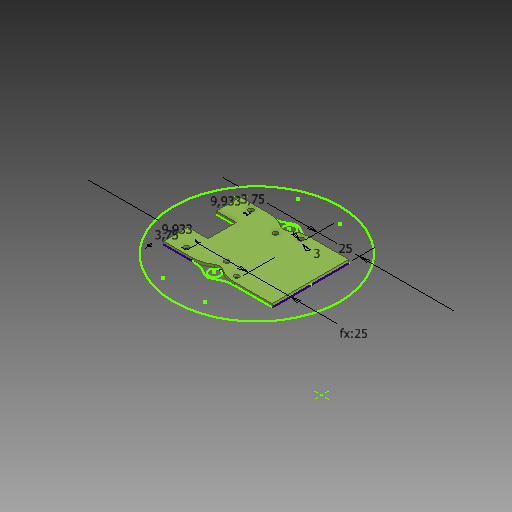
# Autodesk Inventor part: openMV_board
Saved by Autodesk Inventor 2020 (Build 240168000, 168)
## iProperties
Created: 2024-09-29
Part Number: openMV_board
Material: Типовые
Document SubType Name: Modeling
Designer: Ivan
Density: 1 g/cm^3
Appearance: Оливково-зеленый
Author: Ivan
Autodesk Inventor part; units mm, degrees
ref_plane "YZ Plane" through (0, 0, 0) normal (1, 0, 0) x (0, 1, 0)
ref_plane "XZ Plane" through (0, 0, 0) normal (0, 1, 0) x (-1, 0, 0)
ref_plane "XY Plane" through (0, 0, 0) normal (0, 0, 1) x (1, 0, 0)
sketch "Эскиз1" plane through (0, 0, 0) normal (0, 1, 0) x (-1, 0, 0)
  circle A0 centre (22.9, 3.75) radius 1.5
  circle A1 centre (53.2667, -35.05) radius 1.5
  circle A2 centre (22.9, -35.05) radius 1.5
  circle A3 centre (33.4, -38.2774) radius 3.3
  circle A4 centre (33.4, 6.9774) radius 3.3
  circle A5 centre (53.2667, 3.75) radius 1.5
  line L0 (63.2, -24.15) -> (51.2, -24.15)
  line L1 (51.2, -24.15) -> (51.2, -7.15)
  line L2 (51.2, -7.15) -> (63.2, -7.15)
  line L3 (63.2, -7.15) -> (63.2, 7.5)
  line L4 (63.2, 7.5) -> (46.0869, 7.5)
  arc A6 (35.969, 10.672) -> (46.0869, 7.5) centre (46.0869, 25.2227) ccw
  arc A7 (35.969, 10.672) -> (30.831, 10.672) centre (33.4, 6.9774) ccw
  arc A8 (20.7131, 7.5) -> (30.831, 10.672) centre (20.7131, 25.2227) ccw
  line L5 (20.7131, 7.5) -> (-2.1, 7.5)
  line L6 (-2.1, 7.5) -> (-2.1, -38.8)
  line L7 (-2.1, -38.8) -> (20.7131, -38.8)
  arc A9 (30.831, -41.972) -> (20.7131, -38.8) centre (20.7131, -56.5227) ccw
  arc A10 (30.831, -41.972) -> (35.969, -41.972) centre (33.4, -38.2774) ccw
  arc A11 (46.0869, -38.8) -> (35.969, -41.972) centre (46.0869, -56.5227) ccw
  line L8 (46.0869, -38.8) -> (63.2, -38.8)
  line L9 (63.2, -38.8) -> (63.2, -24.15)
  circle A12 centre (30.5522, -15.6437) radius 50
  line L10 (53.2667, -35.05) -> (22.9, -35.05)
  line L11 (53.2667, 3.75) -> (22.9, 3.75)
  point P0 (0, 0)
  point P1 (-2.1, -15.65)
  point P2 (0, 0)
  point P3 (-63.2, 38.8)
  point P4 (63.2, -38.8)
  dimension "d7" = 3.75
  dimension "d8" = 3.75
  dimension "d9" = 9.9333
  dimension "d10" = 9.9333
  dimension "d11" = 25
  dimension "d12" = 25
  dimension "d13" = 3
  constraints: 24 end point, 13 centre point, 12 point on circle, 3 equal radius, 2 horizontal, 8 other
  measures "d7" distance from line of L8 L10.start
  measures "d8" distance from line of L4 L11.start
  measures "d9" distance from line of L3 L11.start
  measures "d10" distance from line of L9 L10.start
  measures "d11" distance from line of L6 L10.end
  measures "d12" distance from line of L6 L11.end
  measures "d13" diameter of A2
sketch "Эскиз2" plane through (0, 0, 0) normal (0, 1, 0) x (-1, 0, 0)
  line L0 (63.2, 7.5) -> (-2.1, 7.5)
  line L1 (-2.1, 7.5) -> (-2.1, -38.8)
  line L2 (-2.1, -38.8) -> (63.2, -38.8)
  line L3 (63.2, -38.8) -> (63.2, 7.5)
  arc A0 (35.969, 10.672) -> (46.0869, 7.5) centre (46.0869, 25.2227) ccw projected
  arc A1 (35.969, 10.672) -> (30.831, 10.672) centre (33.4, 6.9774) ccw projected
  arc A2 (20.7131, 7.5) -> (30.831, 10.672) centre (20.7131, 25.2227) ccw projected
  arc A3 (46.0869, -38.8) -> (35.969, -41.972) centre (46.0869, -56.5227) ccw projected
  arc A4 (30.831, -41.972) -> (35.969, -41.972) centre (33.4, -38.2774) ccw projected
  arc A5 (30.831, -41.972) -> (20.7131, -38.8) centre (20.7131, -56.5227) ccw projected
  arc A6 (46.0869, 7.5) -> (35.969, 4.328) centre (46.0869, -10.2227) ccw
  arc A7 (30.831, 4.328) -> (35.969, 4.328) centre (33.4, 8.0226) ccw
  arc A8 (30.831, 4.328) -> (20.7131, 7.5) centre (20.7131, -10.2227) ccw
  arc A9 (35.969, -35.628) -> (46.0869, -38.8) centre (46.0869, -21.0773) ccw
  arc A10 (35.969, -35.628) -> (30.831, -35.628) centre (33.4, -39.3226) ccw
  arc A11 (20.7131, -38.8) -> (30.831, -35.628) centre (20.7131, -21.0773) ccw
  circle A12 centre (53.2667, 3.75) radius 1.5 projected
  circle A13 centre (53.2667, -35.05) radius 1.5 projected
  circle A14 centre (22.9, -35.05) radius 1.5 projected
  circle A15 centre (22.9, 3.75) radius 1.5 projected
  line L4 (51.2, -7.15) -> (63.2, -7.15) projected
  line L5 (51.2, -24.15) -> (51.2, -7.15) projected
  line L6 (63.2, -24.15) -> (51.2, -24.15) projected
  line L7 (49.7, 2.1365) -> (49.6974, -33.4365)
  line L8 (5.237, 2.1365) -> (49.7, 2.1365)
  line L9 (49.6974, -33.4365) -> (5.2344, -33.4365)
  line L10 (5.2344, -33.4365) -> (5.237, 2.1365)
  circle A16 centre (33.6662, -30.3764) radius 1.397
  circle A17 centre (33.6662, -0.9236) radius 1.397
  line L11 (49.7, 2.1365) -> (49.7, -33.4365) construction
  line L12 (49.7, -15.65) -> (51.2, -15.65) construction
  arc A18 (-19.4267, 43.6888) -> (-16.3877, 43.6879) centre (-17.9094, 36.2928) ccw
  circle A19 centre (-3.0489, 41.4072) radius 1.397
  circle A20 centre (-32.5129, 41.4072) radius 1.397
  line L13 (-3.0489, 41.4072) -> (-32.5129, 41.4072)
  line L14 (-17.7809, 41.4072) -> (-17.7809, 38)
  line L15 (30.5522, -15.6437) -> (30.5522, -33.4365) construction
  line L16 (33.6662, -30.3764) -> (33.6662, -0.9236) construction
  dimension "d0" = 35.573
  dimension "d1" = 1.5
  dimension "d4" = 3.0601
  dimension "d5" = 3.0601
  dimension "d6" = 3.114
  constraints: 28 end point, 14 point on circle, 11 centre point, 10 symmetric about line, 4 perpendicular, 3 midpoint, 3 parallel, 2 horizontal, 1 point on line, 1 vertical, 12 other
  measures "d0" distance of L11.start L11.end
  measures "d1" distance of L12.end L12.start
  measures "d4" distance from line of L9 L16.start
  measures "d5" distance from line of L8 L16.end
  measures "d6" distance from line of L16 L15.start
extrude "Выдавливание1" add sketch "Эскиз2" along normal blind 1.6 contours L3 L4 L5 L6 L2 A9 A10 A11 L1 L0 A8 A7 A6 | L7 L9 L10 L8
equation "\"d12\" = d11"
equation "\"d5\" = d4"
